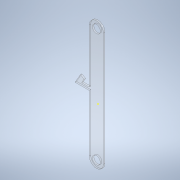
# Autodesk Inventor part: part_0.22 Lexan Intake Arm
Saved by Autodesk Inventor 2021.1 (Build 251245000, 245)
## iProperties
Created: 2021-02-24
Part Number: part_0.22 Lexan Intake Arm
Material: Generic
Document SubType Name: Modeling
Designer: JavDiazV
Density: 1 g/cm^3
Appearance: Polycarbonate - Clear
Author: JavDiazV
Autodesk Inventor part; units mm, degrees
ref_plane "YZ Plane" through (0, 0, 0) normal (1, 0, 0) x (0, 1, 0)
ref_plane "XZ Plane" through (0, 0, 0) normal (0, 1, 0) x (-1, 0, 0)
ref_plane "XY Plane" through (0, 0, 0) normal (0, 0, 1) x (1, 0, 0)
sketch "Sketch1" plane through (0, 0, 0) normal (0, 0, 1) x (1, 0, 0)
  circle A0 centre (0, 235.7819) radius 25.4
  line L0 (-25.4, 235.7819) -> (-25.4, -170.6181)
  circle A1 centre (0, -170.6181) radius 25.4
  line L1 (25.4, -170.6181) -> (25.4, 235.7819)
  line L2 (-25.4, 32.5819) -> (-76.2, 32.5819)
  line L3 (-76.2, 32.5819) -> (-57.15, 65.5775)
  line L4 (-57.15, 65.5775) -> (-43.9135, 57.9354)
  line L5 (-43.9135, 57.9354) -> (-52.4225, 43.1972)
  line L6 (-52.4225, 43.1972) -> (-25.4, 43.1972)
  circle A2 centre (0, 235.7819) radius 14.2875
  circle A3 centre (0, -170.6181) radius 14.2875
  point P0 (0, 0)
  dimension "d52" = 50.8
  dimension "d49" = 50.8
  dimension "d51" = 406.4
  dimension "d53" = 50.8
  dimension "d54" = 38.1
  dimension "d55" = 60
  dimension "d56" = 28.575
  dimension "d57" = 28.575
  constraints: 14 end point, 3 centre point, 3 perpendicular, 2 coincident, 2 point on circle, 2 tangent, 2 vertical, 1 horizontal, 1 midpoint, 1 point on line, 3 other
  measures "d49" diameter of A0
  measures "d51" distance of L0.start L0.end
  measures "d53" distance of L2.start L2.end
  measures "d54" distance of L2.end L3.end
  measures "d55" angle of L2 L3
  measures "d56" diameter of A2
  measures "d57" diameter of A3
sketch "Sketch2" plane through (0, 0, 0) normal (0, 1, 0) x (-1, 0, 0)
  point P0 (0, 0)
extrude "Extrusion8" add sketch "Sketch1" along normal blind 5.588
body "Solid2"
